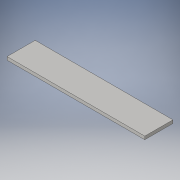
# Autodesk Inventor part: Control pipe holder
Saved by Autodesk Inventor 2016 (Build 200138000, 138)
## iProperties
Created: 2017-01-30
Part Number: Control pipe holder
Material: Generic
Document SubType Name: Modeling
Designer: student1
Density: 1 g/cm^3
Appearance: Default
Mass: 811.16 g
Surface Area: 1448.38 cm^2
Volume: 811.16 cm^3
Author: student1
Autodesk Inventor part; units mm, degrees
ref_plane "YZ Plane" through (0, 0, 0) normal (1, 0, 0) x (0, 1, 0)
ref_plane "XZ Plane" through (0, 0, 0) normal (0, 1, 0) x (-1, 0, 0)
ref_plane "XY Plane" through (0, 0, 0) normal (0, 0, 1) x (1, 0, 0)
sketch "Sketch1" plane through (0, 0, 0) normal (0, 1, 0) x (-1, 0, 0)
  line L0 (302.5767, -33.6533) -> (-154.6233, -33.6533)
  line L1 (-154.6233, -33.6533) -> (-154.6233, -147.9533)
  line L2 (-154.6233, -147.9533) -> (302.5767, -147.9533)
  line L3 (302.5767, -147.9533) -> (302.5767, -33.6533)
  line L4 (-154.6233, -147.9533) -> (-205.4233, -147.9533)
  line L5 (-205.4233, -147.9533) -> (-205.4233, -33.6533)
  line L6 (-205.4233, -33.6533) -> (-154.6233, -33.6533)
  line L7 (-154.6233, -33.6533) -> (-154.6233, -147.9533)
  point P0 (0, 0)
  dimension "d0" = 457.2
  dimension "d1" = 114.3
  dimension "d4" = 50.8
  constraints: 16 end point, 4 parallel, 2 horizontal, 2 perpendicular, 1 point on line
  measures "d0" distance of L1.end L2.end
  measures "d1" distance of L2.end L0.start
  measures "d4" distance of L1.end L4.end
extrude "Extrusion1" add sketch "Sketch1" along normal blind 12.7 contours L3 L2 L1 L0
sketch "Sketch2" plane through (154.6233, 0, -33.6533) normal (1, 0, 0) x (0, 0, -1)
  line L0 (0, 12.7) -> (114.3, 12.7) projected
  line L1 (0, 12.7) -> (114.3, 12.7)
  line L2 (114.3, 12.7) -> (114.3, 0)
  line L3 (114.3, 0) -> (0, 0)
  line L4 (0, 0) -> (0, 12.7)
  point P0 (-33.6533, 0)
  constraints: 8 end point, 2 parallel, 1 horizontal, 1 perpendicular
extrude "Extrusion2" add sketch "Sketch2" along normal blind 50.8
sketch "Sketch3" plane through (205.4233, 0, -33.6533) normal (1, 0, 0) x (0, 0, -1)
  line L0 (114.3, 12.7) -> (0, 12.7) projected
  line L1 (0, 12.7) -> (114.3, 12.7)
  line L2 (114.3, 12.7) -> (114.3, 0)
  line L3 (114.3, 0) -> (0, 0)
  line L4 (0, 0) -> (0, 12.7)
  point P0 (-33.6533, 0)
  constraints: 8 end point, 2 parallel, 1 horizontal, 1 perpendicular
extrude "Extrusion3" add sketch "Sketch3" along normal blind 50.8
body "Solid1"
